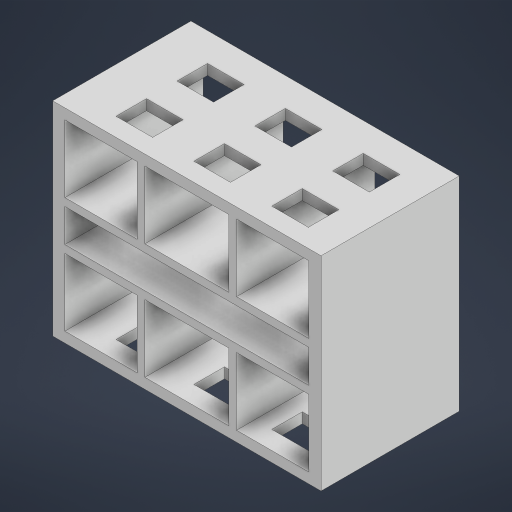
# Autodesk Inventor part: home_templae
Saved by Autodesk Inventor 2024.3 (Build 283343000, 343)
## iProperties
Created: 2025-07-09
Part Number: home_templae
Material: Generic
Document SubType Name: Modeling
Designer: LeoFB
Density: 1 g/cm^3
Appearance: Default
Author: LeoFB
Autodesk Inventor part; units mm, degrees
ref_plane "YZ Plane" through (0, 0, 0) normal (1, 0, 0) x (0, 1, 0)
ref_plane "XZ Plane" through (0, 0, 0) normal (0, 1, 0) x (-1, 0, 0)
ref_plane "XY Plane" through (0, 0, 0) normal (0, 0, 1) x (1, 0, 0)
sketch "Sketch1" plane through (0, 0, 0) normal (0, 0, 1) x (1, 0, 0)
  line L0 (6000, 4500) -> (-6000, 4500)
  line L1 (-6000, 4500) -> (-6000, -4500)
  line L2 (-6000, -4500) -> (6000, -4500)
  line L3 (6000, -4500) -> (6000, 4500)
  line L4 (6000, 4500) -> (-6000, -4500) construction
  line L5 (-6000, 4500) -> (6000, -4500) construction
  line L6 (6600, 5010) -> (-6600, 5010)
  line L7 (-6600, 5010) -> (-6600, -5010)
  line L8 (-6600, -5010) -> (6600, -5010)
  line L9 (6600, -5010) -> (6600, 5010)
  line L10 (6600, 5010) -> (-6600, -5010) construction
  line L11 (-6600, 5010) -> (6600, -5010) construction
  point P0 (0, 0)
  dimension "d0" = 12000
  dimension "d1" = 9000
  dimension "d2" = 13200
  dimension "d3" = 10020
  constraints: 24 end point, 4 midpoint, 4 parallel, 2 horizontal, 2 perpendicular
  measures "d0" distance of L2.end L1.end
  measures "d1" distance of L1.end L0.end
  measures "d2" distance of L8.end L7.end
  measures "d3" distance of L7.end L6.end
extrude "Extrusion1" add sketch "Sketch1" along normal blind 6800
sketch "Sketch2" plane through (-6600, 5010, 0) normal (0, 1, 0) x (1, 0, 0)
  line L0 (11675, -2900) -> (9875, -2900)
  line L1 (9875, -2900) -> (9875, -1400)
  line L2 (9875, -1400) -> (11675, -1400)
  line L3 (11675, -1400) -> (11675, -2900)
  line L4 (13200, 0) -> (13200, -6800) projected
  line L5 (13200, 0) -> (0, 0) projected
  line L6 (11675, -5900) -> (9875, -5900)
  line L7 (9875, -5900) -> (9875, -4400)
  line L8 (9875, -4400) -> (11675, -4400)
  line L9 (11675, -4400) -> (11675, -5900)
  line L10 (7845, -2900) -> (6045, -2900)
  line L11 (6045, -2900) -> (6045, -1400)
  line L12 (6045, -1400) -> (7845, -1400)
  line L13 (7845, -1400) -> (7845, -2900)
  line L14 (7845, -5900) -> (6045, -5900)
  line L15 (6045, -5900) -> (6045, -4400)
  line L16 (6045, -4400) -> (7845, -4400)
  line L17 (7845, -4400) -> (7845, -5900)
  line L18 (4015, -2900) -> (2215, -2900)
  line L19 (2215, -2900) -> (2215, -1400)
  line L20 (2215, -1400) -> (4015, -1400)
  line L21 (4015, -1400) -> (4015, -2900)
  line L22 (4015, -5900) -> (2215, -5900)
  line L23 (2215, -5900) -> (2215, -4400)
  line L24 (2215, -4400) -> (4015, -4400)
  line L25 (4015, -4400) -> (4015, -5900)
  point P0 (6600, 0)
  dimension "d6" = 1800
  dimension "d7" = 1500
  dimension "d8" = 1525
  dimension "d9" = 1400
  dimension "d10" = 1800
  dimension "d11" = 1500
  dimension "d12" = 1500
  dimension "d13" = 1525
  dimension "d14" = 1800
  dimension "d15" = 1500
  dimension "d16" = 1800
  dimension "d17" = 1500
  dimension "d18" = 1500
  dimension "d19" = 1800
  dimension "d20" = 1500
  dimension "d21" = 1800
  dimension "d22" = 1500
  dimension "d23" = 1500
  dimension "d24" = 2030
  dimension "d25" = 2030
  constraints: 48 end point, 12 parallel, 6 horizontal, 6 perpendicular
  measures "d6" distance of L1.end L2.end
  measures "d7" distance of L0.end L1.end
  measures "d8" distance from line of L4 L2.end
  measures "d9" distance from line of L5 L2.end
  measures "d10" distance of L7.end L8.end
  measures "d11" distance of L6.end L7.end
  measures "d12" distance of L8.end L0.start
  measures "d13" distance from line of L4 L8.end
  measures "d14" distance of L11.end L13.start
  measures "d15" distance of L10.end L11.end
  measures "d16" distance of L15.end L16.end
  measures "d17" distance of L14.end L15.end
  measures "d18" distance of L16.end L13.end
  measures "d19" distance of L19.end L21.start
  measures "d20" distance of L18.end L19.end
  measures "d21" distance of L23.end L24.end
  measures "d22" distance of L22.end L23.end
  measures "d23" distance of L24.end L21.end
  measures "d24" distance of L13.start L1.end
  measures "d25" distance of L21.start L11.end
extrude "Extrusion2" cut sketch "Sketch2" against normal blind 11000
sketch "Sketch3" plane through (0, 0, 6800) normal (0, 0, 1) x (1, 0, 0)
  line L0 (6000, 4500) -> (6000, -4500) projected
  line L1 (-6000, -4500) -> (-6000, 4500) projected
  line L2 (6000, 0) -> (7500, 0) construction
  line L3 (-6000, 810) -> (6000, 810)
  line L4 (6000, 810) -> (6000, 1190)
  line L5 (6000, 1190) -> (-6000, 1190)
  line L6 (-6000, 1190) -> (-6000, 810)
  line L7 (6000, 4500) -> (2445, 4500)
  line L8 (-6000, 4500) -> (6000, 4500) projected
  line L9 (2445, 4500) -> (2065, 4500)
  line L10 (2445, 1190) -> (2445, 4500)
  line L11 (2065, 4500) -> (2065, 1190)
  line L12 (-2065, 1190) -> (-2445, 1190)
  line L13 (-2445, 1190) -> (-2445, 4500)
  line L14 (-2445, 4500) -> (-2065, 4500)
  line L15 (-2065, 4500) -> (-2065, 1190)
  line L16 (6000, 0) -> (-6000, 0)
  line L17 (-6000, -810) -> (6000, -810)
  line L18 (6000, -810) -> (6000, -1190)
  line L19 (6000, -1190) -> (-6000, -1190)
  line L20 (-6000, -1190) -> (-6000, -810)
  line L21 (6000, -4500) -> (2445, -4500)
  line L22 (2445, -4500) -> (2065, -4500)
  line L23 (2445, -1190) -> (2445, -4500)
  line L24 (2065, -4500) -> (2065, -1190)
  line L25 (-2065, -1190) -> (-2445, -1190)
  line L26 (-2445, -1190) -> (-2445, -4500)
  line L27 (-2445, -4500) -> (-2065, -4500)
  line L28 (-2065, -4500) -> (-2065, -1190)
  point P0 (6000, 1500)
  point P1 (-2445, 4500)
  point P2 (-6000, 1190)
  point P3 (-6000, 810)
  point P4 (6000, 810)
  point P5 (6000, 1190)
  point P6 (2445, 4500)
  point P7 (2065, 4500)
  point P8 (6000, -1500)
  point P9 (-2445, -4500)
  point P10 (2065, -1190)
  point P11 (2065, 1190)
  dimension "d39" = 3310
  dimension "d46" = 3555
  dimension "d47" = 380
  dimension "d50" = 380
  dimension "d52" = 3555
  dimension "d53" = 0
  dimension "d54" = 0
  constraints: 52 end point, 14 symmetric about line, 5 point on line, 3 horizontal, 3 parallel, 2 midpoint, 2 perpendicular
  measures "d39" distance of L9.end L11.end
  measures "d46" distance between parallel lines of L0 L10
  measures "d47" distance between parallel lines of L10 L11
  measures "d50" distance of L13.end L14.end
  measures "d52" distance between parallel lines of L1 L13
  measures "d53" distance from line of L0 L4.end
  measures "d54" distance between parallel lines of L1 L6
extrude "Extrusion4" add sketch "Sketch3" against normal blind 6800 contours L0 L3 L1 L5 | L10 L5 L11 L8 | L15 L5 L13 L8 | L0 L19 L1 L17 | L23 L22 L24 L19 | L19 L28 L27 L26
body "Solid1"
